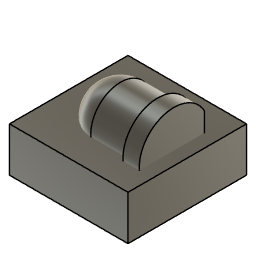
1x1 Jig (Autodesk Fusion 360 design; units mm, degrees)
Autodesk Fusion 360 part; units mm, degrees
note: some values were not read from the file. Set by a fixed rule: which sketch regions a step uses.
box "BoxPrimitive1" add length 16 width 16 height 6 placed x (0, -1, 0) y (1, 0, 0) z (0, 0, 1) at (0, 0, 0) makes body 1
ref_plane "WorkPlane1" through (12, -8, 3) normal (1, 0, 0) x (0, 0, 1)
sketch "Sketch7" plane through (12, -8, 3) normal (1, 0, 0) x (0, 1, 0)
  line L0 (0, 0) -> (0, 3.35)
  circle A0 centre (0, 3.35) radius 4.675
  line L1 (-4.675, 3.35) -> (4.125, 3.35)
  line L2 (4.125, 3.35) -> (4.125, 1.15)
  line L3 (4.125, 3.35) -> (4.125, 5.55)
  circle A1 centre (0, 3.35) radius 4.025
  dimension "d24" = 3.35
  dimension "d25" = 9.35
  dimension "d26" = 8.8
  dimension "d29" = 8.05
  constraint coincident L0.start origin
  constraint vertical L0
  constraint coincident L0.end A0.centre
  constraint coincident A0 L1.start
  constraint perpendicular L0 L1
  constraint coincident A0 L2.end
  constraint perpendicular L1 L2
  constraint coincident A0 L3.end
  constraint perpendicular L1 L3
  constraint concentric A0 A1
  measures "d24" distance of L0.start L0.end
  measures "d25" diameter of A0
  measures "d26" distance of L1.start L1.end
  measures "d29" diameter of A1
extrude "Extrude6" add sketch "Sketch7" along normal blind 2.2 separate body contours A0 L1 L3 A1 | A0 L1 L2 A1 | L1 A1 | L1 A1 makes body 2
extrude "Extrude7" add sketch "Sketch7" against normal blind 9 separate body contours L1 A1 | L1 A1 makes body 3
fillet "Fillet4" radius 4 1 edges at (3, -11.7526, 7.8055) on bodies 3
